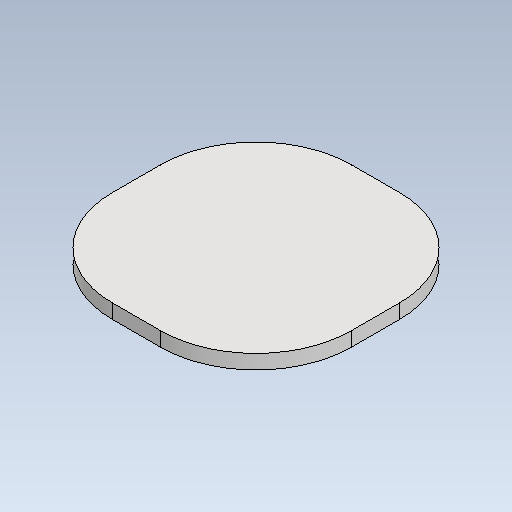
# Autodesk Inventor part: power-bank-bump
Saved by Autodesk Inventor 2025 (Build 290162000, 162)
## iProperties
Created: 2025-08-23
Part Number: power-bank-bump
Material: Generic
Document SubType Name: Modeling
Designer: HP
Density: 1 g/cm^3
Appearance: Default
Author: HP
Autodesk Inventor part; units mm, degrees
ref_plane "YZ Plane" through (0, 0, 0) normal (1, 0, 0) x (0, 1, 0)
ref_plane "XZ Plane" through (0, 0, 0) normal (0, 1, 0) x (-1, 0, 0)
ref_plane "XY Plane" through (0, 0, 0) normal (0, 0, 1) x (1, 0, 0)
sketch "Sketch1" plane through (0, 0, 0) normal (0, 1, 0) x (-1, 0, 0)
  line L0 (15, -15) -> (-35, -15)
  line L1 (-35, -15) -> (-35, 35)
  line L2 (-35, 35) -> (15, 35)
  line L3 (15, 35) -> (15, -15)
  line L4 (15, -15) -> (-35, 35) construction
  line L5 (-35, -15) -> (15, 35) construction
  point P0 (-10, 10)
  dimension "d2" = 50
  dimension "d3" = 50
  constraints: 12 end point, 2 midpoint, 2 parallel, 1 horizontal, 1 perpendicular
  measures "d2" distance of L1.end L2.end
  measures "d3" distance of L0.end L1.end
extrude "Extrusion1" add sketch "Sketch1" along normal blind 3
fillet "Fillet1" radius 20 4 edges at (35, 1.5, 35) (-15, 1.5, 35) (-15, 1.5, -15) (35, 1.5, -15)
equation "\"d2\" = d3"
body "Solid1"
